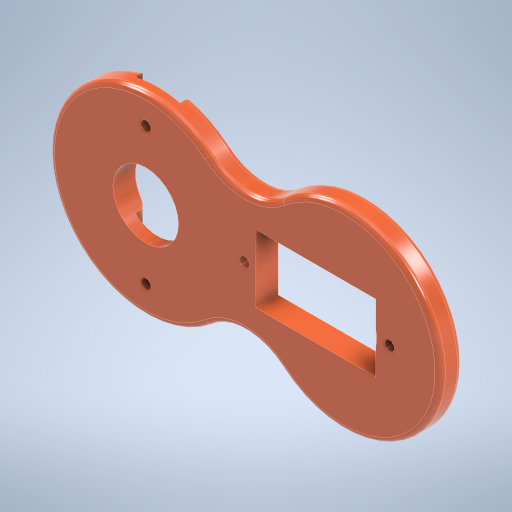
# Autodesk Inventor part: firsarm
Saved by Autodesk Inventor 2023.2 (Build 272271000, 271)
## iProperties
Created: 2022-12-18
Part Number: firsarm
Material: Polystyrene
Document SubType Name: Modeling
Designer: omrfrkmll
Density: 1.021 g/cm^3
Appearance: Smooth - Light Orange
Author: omrfrkmll
Autodesk Inventor part; units mm, degrees
ref_plane "YZ Plane" through (0, 0, 0) normal (1, 0, 0) x (0, 1, 0)
ref_plane "XZ Plane" through (0, 0, 0) normal (0, 1, 0) x (-1, 0, 0)
ref_plane "XY Plane" through (0, 0, 0) normal (0, 0, 1) x (1, 0, 0)
sketch "Sketch2" plane through (0, 0, 0) normal (0, 0, 1) x (1, 0, 0)
  circle A0 centre (0, 0) radius 18.5
  circle A1 centre (38, 0) radius 6.3
  circle A2 centre (0, 0) radius 6.3
  circle A3 centre (38, 0) radius 18.5
  line L0 (-1.1534, 0) -> (34.5511, 0)
  arc A4 (12.005, 14.0759) -> (25.995, 14.0759) centre (19, 22.2775) ccw
  arc A5 (25.995, -14.0759) -> (12.005, -14.0759) centre (19, -22.2775) ccw
  line L1 (1.1428, -18.5) -> (0, -18.5)
  line L2 (1.1428, 18.5) -> (0, 18.5)
  point P0 (38, 18.5)
  point P1 (38, -18.5)
  point P2 (18.5, 0)
  dimension "d0" = 37
  dimension "d19" = 12.6
  dimension "d20" = 37
  dimension "d26" = 38
  constraints: 11 point on circle, 6 centre point, 6 end point, 4 tangent, 3 symmetric about line, 1 coincident, 1 equal radius, 1 horizontal, 1 point on line, 1 other
  measures "d0" diameter of A0
  measures "d19" diameter of A2
  measures "d20" diameter of A3
  measures "d26" distance of A1.centre point (0, 0)
extrude "Extrusion1" add sketch "Sketch2" along normal blind 4.3
sketch "Sketch3" plane through (0, 0, 4.3) normal (0, 0, 1) x (1, 0, 0)
  circle A0 centre (38, 0) radius 6.3 projected
  line L0 (38, 0) -> (38, 2.8384)
  point P0 (0, 0)
  point P1 (46.7, 0)
  point P2 (18.9, 0)
  dimension "d7" = 27.8
  dimension "d16" = 8.7
  constraints: 2 end point, 1 vertical
  measures "d7" distance of point (46.7, 0) point (18.9, 0)
  measures "d16" distance of L0.start point (46.7, 0)
hole "Hole1" at (46.7, 0, 4.3) at (18.9, 0, 4.3) direction (0, 0, -1) diameter 2 depth 7
sketch "Sketch4" plane through (0, 0, 0) normal (0, 0, -1) x (-1, 0, 0)
  circle A0 centre (0, 0) radius 6.3 projected
  line L0 (0, 3.334) -> (0, -2.474)
  line L1 (-2.132, 0) -> (2.0257, 0)
  line L2 (-4.2951, 19.0635) -> (4.2951, 19.0635)
  line L3 (4.2951, 19.0635) -> (4.2951, -19.0635)
  line L4 (4.2951, -19.0635) -> (-4.2951, -19.0635)
  line L5 (-4.2951, -19.0635) -> (-4.2951, 19.0635)
  point P0 (4.2951, -4.609)
  point P1 (-4.2951, -4.609)
  point P2 (-4.2951, 4.609)
  point P3 (4.2951, 4.609)
  constraints: 12 end point, 2 horizontal, 2 parallel, 2 point on line, 1 perpendicular, 1 vertical, 2 other
extrude "Extrusion2" cut sketch "Sketch4" against normal blind 2 contours A0 L5 L2 L3 | L3 L4 L5 A0
sketch "Sketch5" plane through (0, 0, 4.3) normal (0, 0, 1) x (1, 0, 0)
  circle A0 centre (38, 0) radius 6.3 projected
  line L0 (38, 0) -> (38, 11.0593)
  line L1 (38, 0) -> (42.2148, 0)
  line L2 (21.1, 6.5) -> (44.1, 6.5)
  line L3 (44.1, 6.5) -> (44.1, -6.5)
  line L4 (44.1, -6.5) -> (21.1, -6.5)
  line L5 (21.1, -6.5) -> (21.1, 6.5)
  circle A1 centre (46.7, 0) radius 1 projected
  point P0 (0, 0)
  point P1 (44.1, -1.5748)
  point P2 (44.1, 1.5748)
  dimension "d21" = 13
  dimension "d22" = 23
  dimension "d23" = 2.6
  constraints: 12 end point, 2 horizontal, 2 parallel, 1 perpendicular, 1 vertical, 1 other
  measures "d21" distance between parallel lines of L4 L2
  measures "d22" distance between parallel lines of L3 L5
  measures "d23" distance from line of L3 A1.centre
extrude "Extrusion3" cut sketch "Sketch5" against normal blind 4.3 contours A0 L0 L2 L3 | L3 L4 L5 L2 L0 A0
fillet "Fillet1" radius 1 14 edges at (19, 11.498, 0) (8.3822, 16.4921, 0) (19, -11.498, 0) (8.3822, -16.4921, 0) (56.5, 0, 0) (-18.5, 0, 0) (19, -11.498, 4.3) (56.5, 0, 4.3) (19, 11.498, 4.3) (-18.5, 0, 4.3) (4.2951, 11.3017, 0) (4.2951, -11.3017, 0) (-4.2951, 11.3017, 0) (-4.2951, -11.3017, 0)
sketch "Sketch7" plane through (0, 0, 2) normal (0, 0, -1) x (-1, 0, 0)
  circle A0 centre (0, 0) radius 6.3 projected
  line L0 (0, 0) -> (0, 23.1769)
  line L1 (0, 0) -> (3.1147, 0)
  point P0 (0, 13.1)
  point P1 (0, -13.1)
  dimension "d28" = 26.2
  constraints: 4 end point, 2 point on line, 1 horizontal, 1 symmetric about line, 1 vertical
  measures "d28" distance of point (0, -13.1) point (0, 13.1)
hole "Hole2" at (0, 13.1, 2) at (0, -13.1, 2) direction (0, 0, 1) diameter 2 depth 2.3
body "Solid1"
